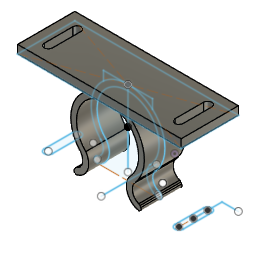
gancio supporto pompa piscina (Autodesk Fusion 360 design; units mm, degrees)
Autodesk Fusion 360 part; units mm, degrees
sketch "Schizzo1" plane through (0, 0, 0) normal (0, 0, 1) x (1, 0, 0)
  arc A0 through (-18.6566, -28.6062, 0) (-12.069, -28.6062, 6.1446) (-13.3278, -28.6062, 15.0648)
  arc A1 through (18.779, -28.6062, 16.2126) (-1.5952, -28.6062, 51.0495) (-16.8373, -28.6062, 13.6811)
  arc A2 through (13.7434, -28.6062, 15.4867) (-0.2961, -28.6062, 47.6039) (-13.3278, -28.6062, 15.0648)
  arc A3 through (-19.1018, -28.6062, 3.6283) (-15.3035, -28.6062, 7.8354) (-16.5512, -28.6062, 13.3645)
  line L0 (-20.3329, -28.6062, 2.2348) -> (-19.8514, -28.6062, 3.0129)
  arc A4 through (-19.1018, -28.6062, 3.6283) (-19.5277, -28.6062, 3.3828) (-19.8514, -28.6062, 3.0129)
  arc A5 through (-20.3329, -28.6062, 2.2348) (-20.2573, -28.6062, 0.5454) (-18.6566, -28.6062, 0)
  line L1 (-16.8373, -28.6062, 13.6811) -> (-16.5512, -28.6062, 13.3645)
  line L2 (0, -28.6062, 28.6062) -> (0, -28.6062, 4.6062)
  line L3 (16.8373, -28.6062, 13.6811) -> (16.5512, -28.6062, 13.3645)
  line L4 (20.3329, -28.6062, 2.2348) -> (19.8514, -28.6062, 3.0129)
  arc A6 through (16.5512, -28.6062, 13.3645) (15.3035, -28.6062, 7.8354) (19.1018, -28.6062, 3.6283)
  arc A7 through (13.3278, -28.6062, 15.0648) (12.069, -28.6062, 6.1446) (18.6566, -28.6062, 0)
  arc A8 through (19.8514, -28.6062, 3.0129) (19.5277, -28.6062, 3.3828) (19.1018, -28.6062, 3.6283)
  arc A9 through (18.6566, -28.6062, 0) (20.2573, -28.6062, 0.5454) (20.3329, -28.6062, 2.2348)
  line L5 (18.779, -28.6062, 16.2126) -> (16.8373, -28.6062, 13.6811)
  line L6 (13.7434, -28.6062, 15.4867) -> (13.3278, -28.6062, 15.0648)
  line L7 (-19.0573, -28.6062, -0.0545) -> (19.0573, -28.6062, -0.0545)
  line L8 (0, -28.6062, 28.6062) -> (0, -28.6062, 51)
  line L9 (0, -28.6062, 51) -> (15, -28.6062, 51)
  line L10 (15, -28.6062, 51) -> (15, -28.6062, 45.3767)
  line L11 (0, -28.6062, 51) -> (-15, -28.6062, 51)
  line L12 (-15, -28.6062, 51) -> (-15, -28.6062, 45.3767)
  line L13 (-50, -46.1062, 51) -> (50, -46.1062, 51)
  line L14 (50, -46.1062, 51) -> (50, -11.1062, 51)
  line L15 (50, -11.1062, 51) -> (-50, -11.1062, 51)
  line L16 (-50, -11.1062, 51) -> (-50, -46.1062, 51)
  line L17 (-50, -46.1062, 51) -> (50, -11.1062, 51) construction
  line L18 (50, -46.1062, 51) -> (-50, -11.1062, 51) construction
  line L19 (50, -11.1) -> (40, -11.1)
  line L20 (40, -11.1) -> (40, -28.6)
  line L21 (42.5, -37.35) -> (42.5, -19.85)
  arc A10 (42.5, -19.85) -> (37.5, -19.85) centre (40, -19.85) ccw
  line L22 (37.5, -19.85) -> (37.5, -37.35)
  arc A11 (37.5, -37.35) -> (42.5, -37.35) centre (40, -37.35) ccw
  line L23 (40, -37.35) -> (40, -19.85) construction
  line L24 (0, -45) -> (0, -11.1754)
  line L25 (-42.5, -37.35) -> (-42.5, -19.85)
  arc A12 (-42.5, -37.35) -> (-37.5, -37.35) centre (-40, -37.35) ccw
  line L26 (-37.5, -19.85) -> (-37.5, -37.35)
  arc A13 (-37.5, -19.85) -> (-42.5, -19.85) centre (-40, -19.85) ccw
  point P0 (0, -28.6062)
  point P1 (0, -28.6062)
  point P2 (40, -28.6)
  dimension "d1" = 38
  dimension "d2" = 45
  dimension "d9" = 1.5
  dimension "d24" = 15
  dimension "d25" = 15
  dimension "d29" = 100
  dimension "d30" = 35
  dimension "d34" = 10
  dimension "d35" = 17.5
  dimension "d36" = 5
  constraint coincident origin P1
  constraint coincident P0 P1
  constraint coincident P1 P0
  constraint horizontal L19
  constraint perpendicular L19 L20
  constraint tangent L21 A10
  constraint tangent A10 L22
  constraint parallel L21 L22
  constraint tangent L22 A11
  constraint tangent L21 A11
  constraint parallel L20 L23
  constraint coincident P2 L20.end
  constraint midpoint L23 P2
  constraint vertical L24
  constraint symmetric L21.start L24 L25.start
  constraint symmetric L21.end L24 L25.end
  constraint symmetric A10.end L24 L26.start
  constraint symmetric L22.end L24 A12.end
  constraint symmetric A10 L24 A13
  constraint symmetric A11 L24 A12
  measures "d34" distance of L19.start L19.end
  measures "d35" distance of L19.end P2
  measures "d36" diameter of A10
extrude "Estrusione3" add sketch "Schizzo1" along normal mid plane 25 contours A0 A1 A2 A3 L0 A4 A5 L1 L8 L11 | A1 A2 L3 L4 A6 A7 A8 A9 L5 L6 L8 L9 | A1 L9 L11 in plane through (0, -28.6062, 0) normal (0, 1, 0)
extrude "Estrusione5" add sketch "Schizzo1" along normal mid plane 25 contours A1 L9 L10 | A1 L11 L12 in plane through (0, -28.6062, 0) normal (0, 1, 0)
extrude "Estrusione6" add sketch "Schizzo1" along normal blind 5 contours L13 L14 L15 L16 in plane through (0, 0, 51) normal (0, 0, 1)
extrude "Estrusione7" cut sketch "Schizzo1" along normal blind 70
equation "d35 = ( 35 / 2 ) * 1 mm"
